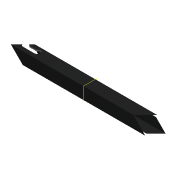
# Autodesk Inventor part: KozepsoOsszekotok
Saved by Autodesk Inventor 2015 SP1 (Build 190203100, 203)
## iProperties
Created: 2014-09-27
Part Number: KozepsoOsszekotok
Material: Steel, Alloy
Document SubType Name: Modeling
Designer: laca
Density: 7.73 g/cm^3
Appearance: Semi-Polished
Mass: 233.54 g
Surface Area: 407.192 cm^2
Volume: 30.2122 cm^3
Author: laca
Autodesk Inventor part; units mm, degrees
ref_plane "YZ Plane" through (0, 0, 0) normal (1, 0, 0) x (0, 1, 0)
ref_plane "XZ Plane" through (0, 0, 0) normal (0, 1, 0) x (-1, 0, 0)
ref_plane "XY Plane" through (0, 0, 0) normal (0, 0, 1) x (1, 0, 0)
derived "KétvégenMartSzelvény.ipt"
sketch "Sketch1" plane through (0, 0, 0) normal (1, 0, 0) x (0, 1, 0)
  line L0 (0, 0) -> (12, 0)
  line L1 (12, 0) -> (12, 12)
  line L2 (12, 12) -> (0, 12)
  line L3 (0, 12) -> (0, 0)
  line L4 (-1.5, 13.5) -> (13.5, 13.5)
  line L5 (13.5, 13.5) -> (13.5, -1.5)
  line L6 (13.5, -1.5) -> (-1.5, -1.5)
  line L7 (-1.5, -1.5) -> (-1.5, 13.5)
extrude "Extrusion1" add sketch "Sketch1" along normal blind 190
sketch "Sketch3" plane through (0, -1.5, -1.5) normal (0, -1, 0) x (1, 0, 0)
  arc A0 (13.094, 10) -> (13.094, 5) centre (13.094, 7.5) ccw
  arc A1 (28.094, 5) -> (28.094, 10) centre (28.094, 7.5) ccw
  line L0 (0, 15) -> (190, 15) projected
  line L1 (0, 0) -> (190, 0) projected
  line L2 (0, 0) -> (0, 15) projected
  line L3 (13.094, 10) -> (28.094, 10)
  line L4 (13.094, 5) -> (28.094, 5)
  point P0 (0, 1.5)
  dimension "d7" = 5
  dimension "d10" = 5
  dimension "d11" = 7.5
  dimension "d14" = 15
  dimension "d16" = 7.5
  dimension "d17" = 15
  dimension "d18" = 13.094
  constraints: 4 end point, 4 point on circle, 2 centre point, 2 tangent, 1 horizontal
  measures "d7" diameter of A0
  measures "d10" diameter of A1
  measures "d11" distance from line of L0 A0.centre
  measures "d14" distance between parallel lines of L1 L0
  measures "d16" distance from line of L0 A1.centre
  measures "d17" distance of A1.centre A0.centre
  measures "d18" distance from line of L2 A0.centre
extrude "Extrusion2" cut sketch "Sketch3" against normal through all
ref_plane "Work Plane1" through (95, -1.5, 13.5) normal (-1, 0, 0) x (0, 0, 1)
sketch "Sketch4" plane through (0, -1.5, -1.5) normal (0, -1, 0) x (1, 0, 0)
  point P0 (28.4, 6.4696)
  point P1 (13.4, 6.4696)
hole "Hole1" at (28.4, -1.5, 4.9696) at (13.4, -1.5, 4.9696) direction (0, 1, 0) diameter 6.6 depth 1.5
sketch "Sketch5" plane through (0, 13.5, 13.5) normal (0, 1, 0) x (1, 0, 0)
  point P0 (28.4, 8.5304)
  point P1 (13.4, 8.5304)
hole "Hole3" at (28.4, 13.5, 4.9696) at (13.4, 13.5, 4.9696) direction (0, -1, 0) diameter 6.6 depth 1.5
equation "\"d11\" = 0.5 * d14"
equation "\"d16\" = d11"
body "Solid1"
